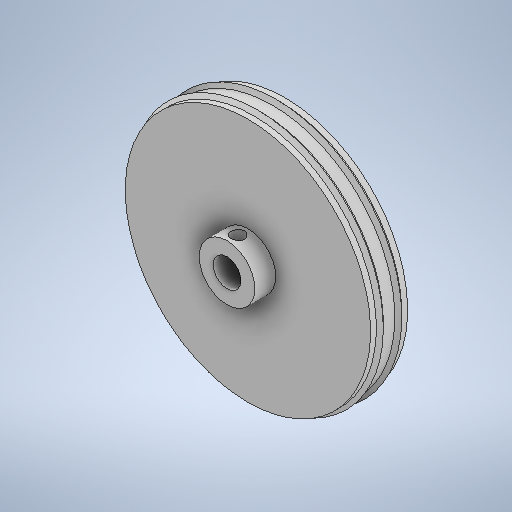
# Autodesk Inventor part: roue
Saved by Autodesk Inventor 2025.2 (Build 292293000, 293)
## iProperties
Created: 2025-03-27
Part Number: roue
Material: Générique
Document SubType Name: Modeling
Designer: enezl
Density: 1 g/cm^3
Appearance: Par défaut
Author: enezl
Autodesk Inventor part; units mm, degrees
ref_plane "YZ Plane" through (0, 0, 0) normal (1, 0, 0) x (0, 1, 0)
ref_plane "XZ Plane" through (0, 0, 0) normal (0, 1, 0) x (-1, 0, 0)
ref_plane "XY Plane" through (0, 0, 0) normal (0, 0, 1) x (1, 0, 0)
sketch "Esquisse1" plane through (0, 0, 0) normal (1, 0, 0) x (0, 1, 0)
  line L0 (35.3, 0) -> (8, 0)
  line L1 (4, -10.66) -> (35.3, -10.66)
  line L2 (35.3, -10.66) -> (35.3, 0) construction
  line L3 (4, 6) -> (8, 6)
  line L4 (8, 6) -> (8, 0)
  line L5 (4, 6) -> (4, -10.66)
  line L6 (0, 31.5501) -> (0, -31.5501)
  line L7 (35.3, -1.665) -> (36.3, -2.665)
  line L8 (36.3, -2.665) -> (35.3, -3.665)
  line L9 (35.3, -5.33) -> (4, -5.33) construction
  line L10 (35.3, -8.995) -> (36.3, -7.995)
  line L11 (36.3, -7.995) -> (35.3, -6.995)
  line L12 (35.3, 0) -> (35.3, -1.665)
  line L13 (35.3, -3.665) -> (35.3, -6.995)
  line L14 (35.3, -8.995) -> (35.3, -10.66)
  point P0 (0, 0)
  dimension "d1" = 10.66
  dimension "d2" = 6
  dimension "d4" = 8
  dimension "d5" = 70.6
  dimension "d6" = 16
  dimension "d7" = 2.665
  dimension "d8" = 135
  dimension "d9" = 1
  constraints: 30 end point, 6 perpendicular, 4 point on line, 3 collinear, 3 symmetric about line, 2 midpoint, 2 vertical, 1 horizontal, 1 parallel, 1 other
  measures "d1" distance of L1.end L0.start
  measures "d2" distance of L0.end L3.end
  measures "d4" diameter of L5 L6
  measures "d5" diameter of L2 L6
  measures "d6" diameter of L4 L6
  measures "d7" vertical distance of L7.end L9.start
  measures "d8" angle of L2 L8
  measures "d9" distance from line of L2 L7.end
revolve "Révolution1" add sketch "Esquisse1" angle 360 about axis through (0, 0, 31.5501) along (0, 0, -1)
sketch "Esquisse2" plane through (0, 0, 0) normal (0, 1, 0) x (-1, 0, 0)
  circle A0 centre (0, 3) radius 1.95
  line L0 (-8, 6) -> (8, 6) projected
  point P0 (0, 0)
  dimension "d11" = 3.9
  dimension "d12" = 3
  constraints: 1 centre point
  measures "d11" diameter of A0
  measures "d12" distance from line of L0 A0.centre
extrude "Extrusion1" cut sketch "Esquisse2" along normal through all
